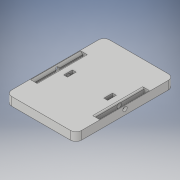
# Autodesk Inventor part: Case Bottom
Saved by Autodesk Inventor 2019 (Build 230136000, 136)
## iProperties
Created: 2022-04-25
Part Number: Case Bottom
Material: Generic
Document SubType Name: Modeling
Designer: Loxei
Density: 1 g/cm^3
Appearance: Default
Author: Loxei
Autodesk Inventor part; units mm, degrees
ref_plane "YZ Plane" through (0, 0, 0) normal (1, 0, 0) x (0, 1, 0)
ref_plane "XZ Plane" through (0, 0, 0) normal (0, 1, 0) x (-1, 0, 0)
ref_plane "XY Plane" through (0, 0, 0) normal (0, 0, 1) x (1, 0, 0)
sketch "Sketch1" plane through (0, 0, 0) normal (0, 1, 0) x (-1, 0, 0)
  line L0 (25, 35) -> (-25, 35)
  line L1 (-25, 35) -> (-25, -35)
  line L2 (-25, -35) -> (25, -35)
  line L3 (25, -35) -> (25, 35)
  line L4 (46.3556, 0) -> (-46.3556, 0) construction
  line L5 (0, 66.4834) -> (0, -66.4834) construction
  point P0 (0, 0)
  dimension "d0" = 70
  dimension "d1" = 50
  constraints: 12 end point, 2 horizontal, 2 midpoint, 2 parallel, 2 perpendicular, 2 symmetric about line, 1 vertical, 2 other
  measures "d0" distance of L2.end L0.start
  measures "d1" distance of L0.start L0.end
extrude "Extrusion1" add sketch "Sketch1" along normal blind 6
fillet "Fillet1" radius 4 4 edges at (25, 3, -35) (-25, 3, -35) (25, 3, 35) (-25, 3, 35)
sketch "Sketch3" plane through (0, 6, 0) normal (0, 1, 0) x (1, 0, 0)
  line L0 (20.8, 17.85) -> (23, 17.85)
  line L1 (23, 17.85) -> (23, -17.85)
  line L2 (23, -17.85) -> (20.8, -17.85)
  line L3 (20.8, -17.85) -> (20.8, 17.85)
  line L4 (25, -31) -> (25, 31) projected
  line L5 (0, 50.4303) -> (0, -42.7858) construction
  point P0 (0, 0)
  dimension "d19" = 2
  dimension "d20" = 2.2
  dimension "d21" = 35.7
  dimension "d22" = 17.85
  constraints: 10 end point, 2 parallel, 1 horizontal, 1 perpendicular, 1 point on line, 1 vertical
  measures "d19" distance between parallel lines of L4 L1
  measures "d20" distance of L0.start L0.end
  measures "d21" distance of L0.end L1.end
  measures "d22" distance from line of L0 point (0, 0)
extrude "Extrusion3" cut sketch "Sketch3" against normal blind 5
sketch "Sketch4" plane through (25, 0, 31) normal (1, 0, 0) x (0, 0, -1)
  circle A0 centre (31, 3.75) radius 1.575
  line L0 (0, 6) -> (62, 6) projected
  line L1 (31, 0) -> (31, 12.876) construction
  dimension "d25" = 3.15
  dimension "d26" = 2.25
  constraints: 2 end point, 1 centre point, 1 point on line, 1 vertical
  measures "d25" diameter of A0
  measures "d26" distance from line of L0 A0.centre
extrude "Extrusion4" cut sketch "Sketch4" against normal blind 12
sketch "Sketch5" plane through (13, 3.75, 0) normal (1, 0, 0) x (0, 0, -1)
  line L0 (-7.2766, 2.25) -> (7.1807, 2.25) construction
  line L1 (-1.65, -2.85) -> (1.65, -2.85)
  line L2 (1.65, -2.85) -> (3.1, 0)
  line L3 (3.1, 0) -> (3.1, 2.25)
  line L4 (-1.65, -2.85) -> (-3.1, 0)
  line L5 (-3.1, 0) -> (-3.1, 2.25)
  line L6 (5.6635, 0) -> (-4.7005, 0) construction
  line L7 (0, 2.25) -> (0, -2.6595) construction
  circle A0 centre (0, 0) radius 1.575 projected
  line L8 (-3.1, 2.25) -> (3.1, 2.25)
  line L9 (31, 2.25) -> (-31, 2.25) projected
  point P0 (0, -3.75)
  point P1 (-37.4528, 45.8008)
  point P2 (-11.2432, 45.8008)
  point P3 (-34.3528, 45.8008)
  point P4 (-40.5528, 45.8008)
  point P5 (0, 2.1)
  dimension "d33" = 6.2
  dimension "d34" = 2.85
  dimension "d35" = 3.3
  constraints: 18 end point, 8 point on line, 2 horizontal, 2 perpendicular, 2 symmetric about line
  measures "d33" distance between parallel lines of L5 L3
  measures "d34" distance from line of L1 A0.centre
  measures "d35" distance of L1.start L1.end
extrude "Extrusion5" cut sketch "Sketch5" along normal blind 2.7
mirror "Mirror1" about plane through (0, 0, 0) normal (1, 0, 0) of "Extrusion3", "Extrusion5", "Extrusion4"
chamfer "Chamfer1" distance 1.6 angle 45 2 edges at (23, 6, 0) (-23, 6, 0)
fillet "Fillet2" radius 1 2 edges at (20.8, 6, 0) (-20.8, 6, 0)
equation "\"d22\" = 0.5 * d21"
equation "\"d26\" = 0.714286 * d25"
body "Solid1"
